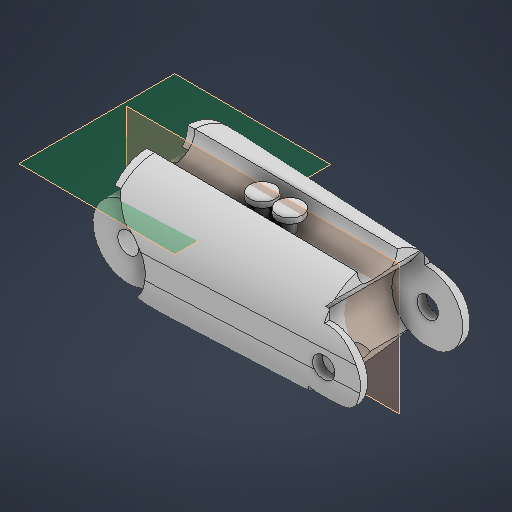
# Autodesk Inventor part: falange2_inidice_V13
Saved by Autodesk Inventor 2026.1 (Build 301233020, 233B)
## iProperties
Created: 2026-01-14
Part Number: falange2_inidice_V13
Material: Generic
Document SubType Name: Modeling
Designer: user
Density: 1 g/cm^3
Appearance: Default
Author: user
Autodesk Inventor part; units mm, degrees
ref_plane "YZ Plane" through (0, 0, 0) normal (1, 0, 0) x (0, 1, 0)
ref_plane "XY Plane" through (0, 0, 0) normal (0, 0, 1) x (1, 0, 0)
sketch "Sketch1" plane through (0, 0, 0) normal (0, 0, 1) x (1, 0, 0)
  line L0 (5.2791, -7.5157) -> (23.7146, -7.6079)
  circle A0 centre (0, 0) radius 1.5
  line L1 (0, 5) -> (0, 9.2)
  circle A1 centre (29, 0) radius 1.5
  arc A2 (26.221, -4.0661) -> (28.5805, 4.9071) centre (29, 0) ccw
  line L2 (28.5805, 4.9071) -> (28.5805, 9.0571)
  line L3 (28.5805, 9.0571) -> (0, 9.2)
  arc A3 (0, 5) -> (2.896, -4.0759) centre (0, 0) ccw
  line L4 (2.896, -4.0759) -> (5.2791, -7.5157)
  line L5 (26.221, -4.0661) -> (23.7146, -7.6079)
  dimension "d13" = 3
  dimension "d36" = 3
  dimension "d37" = 9.85
  dimension "d65" = 0
  dimension "d66" = 29
  dimension "d67" = 4.15
  dimension "d73" = 10
  dimension "d112" = 4.2
  dimension "d144" = 55
  dimension "d172" = 55
  dimension "d173" = 4.339
  dimension "d174" = 4.1846
  constraints: 12 end point, 4 centre point, 4 point on circle, 3 coincident, 2 parallel, 2 vertical
  measures "d13" diameter of A0
  measures "d36" diameter of A1
  measures "d37" diameter of A2
  measures "d65" vertical distance of point (0, 0) A1.centre
  measures "d66" distance of A1.centre point (0, 0)
  measures "d67" distance of L2.start L2.end
  measures "d73" diameter of A3
  measures "d112" distance of L1.start L1.end
  measures "d144" angle of L0 L4
  measures "d172" angle of L0 L5
  measures "d173" distance of L5.start L0.end
  measures "d174" distance of L4.start L0.start
extrude "Extrusion1" add sketch "Sketch1" along normal mid plane 23
sketch "Sketch4" plane through (0, 9.2, -11.5) normal (-1, 0, 0) x (0, 0, 1)
  circle A0 centre (11.5, -13.8108) radius 1.5
  point P0 (11.5, -9.2)
  dimension "d23" = 3
  constraints: 1 centre point
  measures "d23" diameter of A0
extrude "Extrusion4" cut sketch "Sketch4" against normal through all
sketch "Sketch7" plane through (0, 0, 0) normal (0, 0, 1) x (1, 0, 0)
  circle A0 centre (29, 0) radius 5.075
  circle A1 centre (29, 0) radius 1.5 projected
  point P0 (0, 0)
  dimension "d116" = 10.15
  constraints: 1 centre point, 1 coincident
  measures "d116" diameter of A0
extrude "Extrusion6" cut sketch "Sketch7" along normal mid plane 13.41 contours A0 | A1
ref_plane "Work Plane4" through (0, 0, 0) normal (0, 0, 1) x (1, 0, 0)
sketch "Sketch14" plane through (0, 0, 0) normal (0, 0, 1) x (1, 0, 0)
  circle A0 centre (0, 0) radius 5
  dimension "d80" = 10
  constraints: 1 centre point, 1 coincident
  measures "d80" diameter of A0
extrude "Extrusion12" cut sketch "Sketch14" along normal mid plane 3.825
sketch "Sketch39" plane through (5.2791, -7.5157, 11.5) normal (-0.0049999, -0.9999875, 0) x (0.9999875, -0.0049999, 0)
  line L0 (-5.2681, -11.5) -> (20.8531, -11.5)
  line L1 (-5.2681, -2) -> (-27.6718, -2)
  line L2 (-27.6718, -2) -> (-27.6718, -11.5)
  line L3 (-27.6718, -11.5) -> (-5.2681, -11.5)
  line L4 (43.2916, -3.5363) -> (43.3495, -11.742)
  line L5 (43.3495, -11.742) -> (20.8523, -11.6301)
  line L6 (-27.7652, -20.7772) -> (-27.6718, -11.5)
  line L7 (-5.3626, -21) -> (-27.7652, -20.7772)
  line L8 (43.2916, -19.4637) -> (43.3495, -11.742)
  line L9 (23.2182, 0) -> (-5.3626, 0) projected
  line L10 (-5.3626, -23) -> (23.2182, -23) projected
  line L11 (-3.8166, -23) -> (-6.8166, -23) projected
  line L12 (-5.2681, -2) -> (-5.2681, 0)
  line L13 (-5.3626, -21) -> (-5.3626, -23)
  line L14 (-41.6233, -11.5) -> (55.4575, -11.5) projected
  line L15 (23.2382, -4.795) -> (23.2382, -18.205) projected
  line L16 (23.2182, -23) -> (23.2182, 0) projected
  line L17 (23.2182, -11.5) -> (23.2182, -3.5)
  line L18 (-5.3626, -21) -> (43.2992, -18.4461)
  line L19 (-5.2681, -2) -> (43.2992, -4.5539)
  point P0 (-4.1469, -11.0242)
  point P1 (-3.1099, -9.8168)
  point P2 (20.8531, -20)
  point P3 (23.2182, -19.5)
  point P4 (43.2988, -4.5539)
  dimension "d161" = 9.5
  dimension "d162" = -23.963
  dimension "d168" = 0
  dimension "d169" = 8
  constraints: 28 end point, 3 perpendicular, 3 point on line, 3 symmetric about line, 2 horizontal, 2 parallel, 2 vertical alignment, 1 vertical, 3 other
  measures "d161" distance of L0.start L1.start
  measures "d162" horizontal distance of point (-3.11, -9.817) L0.end
  measures "d168" vertical extent of L3
  measures "d169" distance of L17.start L17.end
extrude "Extrusion24" cut sketch "Sketch39" against normal blind 24 contours L3 L2 L1 L19 L16 L14 L0 | L0 L14 L16 L18 L7 L6 L3 | L16 L19 L4 L14 | L14 L15 L5 L16 | L14 L4 L5 L15 | L5 L8 L18 L16 keep common part
fillet "Fillet5" radius 6.7625 2 edges at (14.4968, -7.5618, -8.7348) (14.4968, -7.5618, 8.7383)
fillet "Fillet6" radius 6.7625 2 edges at (14.3375, 9.1283, 8.751) (14.2902, 9.1285, -8.75)
sketch "Sketch12" plane through (0, 0, 11.5) normal (0, 0, 1) x (1, 0, 0)
  circle A0 centre (0, 0) radius 1.5 projected
  circle A1 centre (0, 0) radius 5.075
  dimension "d74" = 10.15
  constraints: 1 centre point, 1 coincident
  measures "d74" diameter of A1
extrude "Extrusion10" cut sketch "Sketch12" against normal blind 4.945
sketch "Sketch13" plane through (0, 0, -11.5) normal (0, 0, -1) x (-1, 0, 0)
  circle A0 centre (0, 0) radius 5.075
  dimension "d77" = 10.15
  constraints: 1 centre point
  measures "d77" diameter of A0
extrude "Extrusion11" cut sketch "Sketch13" against normal blind 4.945
sketch "Sketch16" plane through (0, 0, 0) normal (0, 0, 1) x (1, 0, 0)
  circle A0 centre (0, 0) radius 1.5 projected
  line L0 (-1.9036, 2.4472) -> (1.1675, 2.8722)
  line L1 (1.1675, 2.8722) -> (3.0711, 0.425)
  line L2 (3.0711, 0.425) -> (1.9036, -2.4472)
  line L3 (1.9036, -2.4472) -> (-1.1675, -2.8722)
  line L4 (-1.1675, -2.8722) -> (-3.0711, -0.425)
  line L5 (-3.0711, -0.425) -> (-1.9036, 2.4472)
  dimension "d83" = 5.37
  constraints: 12 end point, 1 coincident, 13 other
  measures "d83" distance between parallel lines of L3 L0
extrude "Extrusion13" cut sketch "Sketch16" along normal mid plane 8.085 contours A0 | L0 L1 L2 L3 L4 L5
ref_plane "Work Plane1" through (0, 9.2, -11.5) normal (0, 1, 0) x (-1, 0, 0)
sketch "Sketch27" plane through (28.5805, 4.9071, -11.5) normal (1, 0, 0) x (0, 0, -1)
  line L0 (0, 4.15) -> (-23, 4.15) projected
  circle A0 centre (-11.5, 4.15) radius 2.8604
  point P0 (-11.5, -4.9071)
  dimension "d117" = 5.7208
  constraints: 1 centre point, 1 midpoint
  measures "d117" diameter of A0
sketch "Sketch28" plane through (0, 9.2, 11.5) normal (0.0049999, 0.9999875, 0) x (0.9999875, -0.0049999, 0)
  line L0 (28.5808, 23) -> (28.5808, 0) projected
  line L1 (28.5808, 11.5) -> (-3.5382, 11.5)
  point P0 (0.046, 11.5)
  constraints: 2 end point, 1 horizontal, 1 midpoint
sweep "Sweep1" cut profiles "Sketch27" path "Sketch28" path curves L1
ref_plane "Work Plane2" through (0, 6.3396, 0) normal (-0.0049999, -0.9999875, 0.0000165) x (0.9999875, -0.0049999, 0)
sketch "Sketch30" plane through (0, 6.3396, 0) normal (-0.0049999, -0.9999875, 0.0000165) x (0.9999875, -0.0049999, 0)
  line L0 (28.5865, 6.7049) -> (28.5865, -6.7051) projected
  line L1 (28.5865, -0.0001) -> (12.3465, -0.0001)
  circle A0 centre (12.3465, -0.0001) radius 0.7321
  point P0 (0.0317, -0.0002)
  dimension "d122" = 16.24
  dimension "d123" = 1.4642
  constraints: 2 end point, 1 centre point, 1 coincident, 1 horizontal, 1 midpoint
  measures "d122" distance of L1.start L1.end
  measures "d123" diameter of A0
extrude "Extrusion19" add sketch "Sketch30" against normal blind 2.1075
sketch "Sketch31" plane through (12.3569, 8.3854, -0.0001) normal (0.0049999, 0.9999875, -0.0000165) x (0.9999875, -0.0049999, 0)
  circle A0 centre (0, 0) radius 0.7321 projected
  circle A1 centre (0, 0) radius 1.774
  point P0 (-12.3148, 0.0001)
  dimension "d126" = 3.548
  constraints: 1 centre point, 1 coincident
  measures "d126" diameter of A1
extrude "Extrusion20" add sketch "Sketch31" along normal up to surface (0.7529 mm away) contours A0 | A1
sketch "Sketch34" plane through (0, 6.3396, 0) normal (-0.0049999, -0.9999875, 0.0000165) x (0.9999875, -0.0049999, 0)
  ellipse E0 centre (28.5665, 0) end of major axis (28.5665, -2.8604) minor radius 0.0143 (28.5675, -2.8536) -> (28.5675, 2.8536) ccw projected
  ellipse E1 centre (-0.0143, 0) end of major axis (-0.0143, -2.8604) minor radius 0.0143 (-0.0143, -2.8604) -> (-0.0143, 2.8604) ccw projected
  line L0 (-0.0143, 0) -> (16.2257, 0)
  circle A0 centre (16.2257, 0) radius 0.7321
  point P0 (0.0317, -0.0002)
  point P1 (0, 2.8604)
  point P2 (0, -2.8604)
  point P3 (-25.0003, -2.8604)
  point P4 (-25.0003, 2.8604)
  dimension "d130" = 16.24
  dimension "d131" = 1.4642
  constraints: 2 end point, 1 centre point, 1 coincident, 1 horizontal, 2 other
  measures "d130" distance of L0.start L0.end
  measures "d131" diameter of A0
extrude "Extrusion21" add sketch "Sketch34" against normal blind 2.1075
sketch "Sketch35" plane through (16.236, 8.366, 0) normal (0.0049999, 0.9999875, -0.0000165) x (0.9999875, -0.0049999, 0)
  circle A0 centre (0, 0) radius 0.7321 projected
  circle A1 centre (0, 0) radius 1.774
  point P0 (-16.194, 0.0002)
  dimension "d134" = 3.548
  constraints: 1 centre point, 1 coincident
  measures "d134" diameter of A1
extrude "Extrusion22" add sketch "Sketch35" along normal up to surface (0.7529 mm away) contours A0 | A1
chamfer "Chamfer1" distance 2 angle 45 1 edges at (28.5805, 5.0576, 0)
chamfer "Chamfer2" distance 2 angle 45 2 edges at (0, 5.075, -7.7588) (0, 5.075, 7.7613)
sketch "Sketch36" plane through (0, 5, -6.555) normal (-1, 0, 0) x (0, 0, 1)
  arc A0 (3.6946, 4.1987) -> (9.4154, 4.1988) centre (6.555, 4.2) ccw projected
  line L0 (14.2162, 2.075) -> (13.11, 2.075) projected
  line L1 (14.1628, 2.131) -> (8.4697, 2.075)
  arc A1 (8.4697, 2.075) -> (9.4154, 4.2) centre (6.555, 4.2) ccw
  arc A2 (6.555, 1.3396) -> (9.4154, 4.2) centre (6.555, 4.2) ccw
  line L2 (6.555, 5.0268) -> (6.555, -0.0494)
  line L3 (-1.047, 2.1319) -> (0, 2.075)
  line L4 (-1.047, 2.1319) -> (4.6403, 2.075)
  arc A3 (3.6946, 4.2) -> (4.6403, 2.075) centre (6.555, 4.2) ccw
  line L5 (0, -10) -> (0, 0) projected
  line L6 (3.9417, -5) -> (10.0382, -5)
  ellipse E0 centre (3.8286, -2.5626) end of major axis (-2.9128, -1.9203) minor radius 6.7625 (3.6946, 4.1987) -> (-1.1013, 2.075) ccw projected
  ellipse E1 centre (9.2863, -2.5626) end of major axis (16.0279, -1.9216) minor radius 6.7625 (14.2162, 2.075) -> (9.4154, 4.1988) ccw projected
  point P0 (6.555, -5)
  point P1 (0, 2.075)
  point P2 (8.4697, 2.075)
  point P3 (0, 2.075)
  point P4 (4.6403, 2.075)
  point P5 (14.2124, 2.075)
  point P6 (9.4154, 4.1988)
  point P7 (3.6946, 4.1987)
  point P8 (3.6946, 4.1987)
  constraints: 8 end point, 7 point on circle, 3 centre point, 2 coincident, 2 concentric, 2 symmetric about line, 1 horizontal, 1 vertical, 8 other
revolve "Revolution1" add sketch "Sketch36" angle 7 about axis through (0, 0, -2.6133) along (0, 0, 1)
equation "\"d13\" = diametroDentroUnion"
equation "\"d36\" = diametroDentroUnion"
equation "\"d73\" = diametroFueraUnion"
equation "\"d80\" = diametroFueraUnion"
equation "\"d16\" = 135deg"
equation "\"d26\" = 135deg"
equation "\"d27\" = 135deg"
equation "\"d30\" = 135deg"
equation "\"d34\" = 23"
equation "\"d35\" = 0"
equation "\"d40\" = 135deg"
equation "\"d41\" = 10.639"
equation "\"d42\" = 11.8875"
equation "\"d43\" = 0"
equation "\"diametroDentroUnion\" = 3"
equation "\"diametroFueraUnion\" = 10"
equation "\"d45\" = 15"
equation "\"d39\" = diametroDentroUnion"
equation "\"tolerancia\" = 0.15"
body "Solid1"
